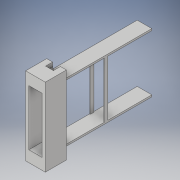
# Autodesk Inventor part: CyberDeckVerticalInsert4
Saved by Autodesk Inventor 2019.4 (Build 234330000, 330)
## iProperties
Created: 2020-08-26
Part Number: CyberDeckVerticalInsert4
Material: Generic
Document SubType Name: Modeling
Designer: Briti
Density: 1 g/cm^3
Appearance: Default
Author: Briti
Autodesk Inventor part; units mm, degrees
ref_plane "YZ Plane" through (0, 0, 0) normal (1, 0, 0) x (0, 1, 0)
ref_plane "XZ Plane" through (0, 0, 0) normal (0, 1, 0) x (-1, 0, 0)
ref_plane "XY Plane" through (0, 0, 0) normal (0, 0, 1) x (1, 0, 0)
sketch "Sketch1" plane through (0, 0, 0) normal (0, 0, 1) x (1, 0, 0)
  line L0 (-13.979, -55.38) -> (13.979, -55.38)
  line L1 (13.979, -55.38) -> (13.979, 55.38)
  line L2 (13.979, 55.38) -> (-13.979, 55.38)
  line L3 (-13.979, 55.38) -> (-13.979, -55.38)
  line L4 (-13.979, -55.38) -> (13.979, 55.38) construction
  line L5 (13.979, -55.38) -> (-13.979, 55.38) construction
  point P0 (0, 0)
  dimension "d0" = 27.958
  dimension "d1" = 110.76
  constraints: 12 end point, 2 midpoint, 2 parallel, 1 horizontal, 1 perpendicular
  measures "d0" distance of L2.end L1.end
  measures "d1" distance of L0.end L1.end
extrude "Extrusion1" add sketch "Sketch1" along normal blind 30
sketch "Sketch2" plane through (0, 0, 0) normal (0, 0, -1) x (-1, 0, 0)
  line L0 (13.979, -55.38) -> (-13.979, -55.38) construction
  line L1 (0, -55.38) -> (0, -49.88) construction
  arc A0 (7.5, -49.88) -> (-7.5, -49.88) centre (0, -49.88) ccw
  line L2 (-7.5, -49.88) -> (-7.5, -55.38)
  line L3 (7.5, -49.88) -> (7.5, -55.38)
  line L4 (-13.979, 55.38) -> (13.979, 55.38) construction
  line L5 (0, 55.38) -> (0, 49.88) construction
  arc A1 (-5.5, 49.88) -> (5.5, 49.88) centre (0, 49.88) ccw
  line L6 (-5.5, 49.88) -> (-5.5, 55.38)
  line L7 (5.5, 49.88) -> (5.5, 55.38)
  line L8 (-5.5, 55.38) -> (5.5, 55.38)
  line L9 (-7.5, -55.38) -> (7.5, -55.38)
  point P0 (0, 0)
  dimension "d4" = 5.5
  dimension "d5" = 15
  dimension "d6" = 5.5
  constraints: 16 end point, 4 perpendicular, 4 point on circle, 4 point on line, 4 tangent, 2 centre point, 2 coincident, 2 collinear, 2 midpoint, 2 vertical
  measures "d4" distance of L1.start L1.end
  measures "d5" diameter of A0
  measures "d6" distance of L5.start L5.end
extrude "Extrusion2" cut sketch "Sketch2" against normal blind 10
sketch "Sketch3" plane through (0, 0, 10) normal (0, 0, -1) x (-1, 0, 0)
  arc A0 (-5.5, 49.88) -> (5.5, 49.88) centre (0, 49.88) ccw projected
  circle A1 centre (0, 49.88) radius 2.4
  arc A2 (7.5, -49.88) -> (-7.5, -49.88) centre (0, -49.88) ccw projected
  circle A3 centre (0, -49.88) radius 2.4
  point P0 (0, 0)
  dimension "d9" = 4.8
  dimension "d10" = 4.8
  constraints: 2 centre point, 2 coincident
  measures "d9" diameter of A1
  measures "d10" diameter of A3
extrude "Extrusion3" cut sketch "Sketch3" against normal blind 10
sketch "Sketch4" plane through (0, 0, 30) normal (0, 0, 1) x (1, 0, 0)
  line L0 (-9.375, -39.5) -> (9.375, -39.5)
  line L1 (9.375, -39.5) -> (9.375, 39.5)
  line L2 (9.375, 39.5) -> (-9.375, 39.5)
  line L3 (-9.375, 39.5) -> (-9.375, -39.5)
  line L4 (-9.375, -39.5) -> (9.375, 39.5) construction
  line L5 (9.375, -39.5) -> (-9.375, 39.5) construction
  point P0 (0, 0)
  dimension "d13" = 18.75
  dimension "d14" = 79
  constraints: 12 end point, 2 midpoint, 2 parallel, 1 horizontal, 1 perpendicular
  measures "d13" distance of L2.end L1.end
  measures "d14" distance of L1.end L0.end
extrude "Extrusion4" cut sketch "Sketch4" against normal blind 30
sketch "Sketch5" plane through (0, 0, 0) normal (0, 0, -1) x (-1, 0, 0)
  line L0 (9.375, -39.5) -> (-9.375, -39.5) construction
  line L1 (-9.375, -39.5) -> (-10.375, -39.5) construction
  line L2 (9.375, -39.5) -> (10.375, -39.5) construction
  line L3 (-10.375, -39.5) -> (10.375, -39.5)
  line L4 (10.375, -39.5) -> (10.375, -42)
  line L5 (10.375, -42) -> (-10.375, -42)
  line L6 (-10.375, -42) -> (-10.375, -39.5)
  line L7 (-9.375, -39.5) -> (-9.375, 39.5) construction
  line L8 (-9.375, 39.5) -> (-10.375, 39.5) construction
  line L9 (-9.375, 39.5) -> (9.375, 39.5) construction
  line L10 (9.375, 39.5) -> (10.375, 39.5) construction
  line L11 (-10.375, 39.5) -> (10.375, 39.5)
  line L12 (10.375, 39.5) -> (10.375, 42)
  line L13 (10.375, 42) -> (-10.375, 42)
  line L14 (-10.375, 42) -> (-10.375, 39.5)
  point P0 (0, 0)
  dimension "d17" = 1
  dimension "d18" = 1
  dimension "d19" = 2.5
  dimension "d20" = 1
  dimension "d21" = 1
  dimension "d22" = 2.5
  constraints: 24 end point, 4 horizontal, 4 parallel, 2 collinear, 2 perpendicular
  measures "d17" distance of L0.end L1.end
  measures "d18" distance of L0.start L2.end
  measures "d19" distance of L2.end L4.end
  measures "d20" distance of L7.end L8.end
  measures "d21" distance of L9.end L10.end
  measures "d22" distance of L12.end L10.end
extrude "Extrusion5" add sketch "Sketch5" along normal blind 125
sketch "Sketch6" plane through (-9.375, 39.5, 30) normal (0, -1, 0) x (1, 0, 0)
  line L0 (19.75, -30) -> (-1, -30) construction
  line L1 (19.75, -30) -> (19.75, -155) construction
  line L2 (19.75, -30) -> (19.75, -155) construction
  line L3 (19.75, -30) -> (19.75, -155) projected
  line L4 (19.75, -92.5) -> (18.75, -92.5)
  line L5 (18.75, -92.5) -> (18.75, -87.5)
  line L6 (18.75, -87.5) -> (19.75, -87.5)
  line L7 (19.75, -87.5) -> (19.75, -92.5)
  line L8 (-1, -30) -> (-1, -155) projected
  line L9 (-1, -92.5) -> (0, -92.5)
  line L10 (0, -92.5) -> (0, -87.5)
  line L11 (0, -87.5) -> (-1, -87.5)
  line L12 (-1, -87.5) -> (-1, -92.5)
  point P0 (9.375, -30)
  dimension "d25" = 1
  dimension "d26" = 5
  dimension "d27" = 1
  dimension "d28" = 5
  constraints: 18 end point, 4 parallel, 2 horizontal, 2 midpoint, 2 perpendicular, 1 vertical
  measures "d25" distance of L5.end L6.end
  measures "d26" distance of L4.end L5.end
  measures "d27" distance of L11.end L10.end
  measures "d28" distance of L10.end L9.end
extrude "Extrusion6" add sketch "Sketch6" along normal blind 80
body "Solid1"
